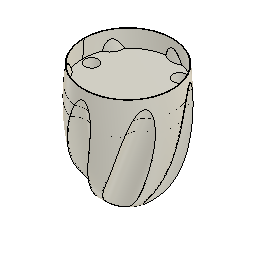
minlampshade twist tall v5 (Autodesk Fusion 360 design; units mm, degrees)
Autodesk Fusion 360 part; units mm, degrees
sketch "Sketch1" plane through (0, 0, 0) normal (0, 1, 0) x (1, 0, 0)
  line L0 (-68, -178) -> (68, -178)
  line L1 (68, -178) -> (68, 0)
  line L2 (-68, 0) -> (-68, -178)
  line L3 (-68, 0) -> (0, 0)
  line L4 (0, 0) -> (68, 0)
  spline S0 degree 5 poles (-68, -178) (-69.3462, -164.4991) (-71.1864, -138.6764) (-71.3876, -103.4793) (-66.4744, -63.741) (-51.543, -26.8671) (-28.7199, -3.9358) (0, 3.9151) (28.7199, -3.9358) (51.543, -26.8671) (66.4744, -63.741) (71.3876, -103.4793) (71.1864, -138.6764) (69.3462, -164.4991) (68, -178) knots 0 0 0 0 0 0 0.1 0.2 0.3 0.4 0.5 0.6 0.7 0.8 0.9 1 1 1 1 1 1
  line L5 (-10, 0) -> (10, 0)
  line L6 (-68, -8) -> (68, -8)
  line L7 (-27.7683, -8) -> (27.7683, -8)
  line L8 (27.7683, -8) -> (27.7683, 0)
  line L9 (27.7683, 0) -> (-27.7683, 0)
  line L10 (-27.7683, 0) -> (-27.7683, -8)
  line L11 (0, -178) -> (0, 0)
  dimension "d2" = 136
  dimension "d4" = 170
  dimension "d5" = 8
  dimension "d6" = 55.5365
  constraint horizontal L0
  constraint vertical L1
  constraint vertical L2
  constraint perpendicular L2 L3
  constraint perpendicular L1 L4
  constraint coincident L3.end L4.start
  constraint equal L3 L4
  constraint coincident L3 L4.start
  constraint midpoint L3.end L5
  constraint coincident L4 L5.end
  constraint coincident L2 L6.start
  constraint coincident L1 L6.end
  constraint perpendicular L1 L6
  constraint horizontal L7
  constraint vertical L8
  constraint horizontal L9
  constraint vertical L10
  constraint coincident L4 L8.end
  constraint coincident S0 L7.start
  constraint coincident L6 L7.start
  constraint coincident S0 L7.end
  constraint midpoint L0 L11.start
  measures "d2" distance of L0.start L0.end
  measures "d4" distance of L0 L6
  measures "d5" distance of L3 L6
  measures "d6" distance of L8 L10
revolve "Revolve1" add sketch "Sketch1" angle 360 about axis through (0, 0, 178) along (0, 0, -1) contours L0 L2 S0 L6 L7 L11 | L2 S0 makes body 1
sketch "Sketch2" plane through (0, 0, 8) normal (0, 0, -1) x (1, 0, 0)
  circle A0 centre (0, 0) radius 27.7683
  circle A1 centre (0, 0) radius 15
  dimension "d8" = 30
  constraint concentric A0 A1
  measures "d8" diameter of A1
extrude "Extrude1" cut sketch "Sketch2" against normal up to surface (170 mm away) contours A1 bodies 1
sketch "Sketch3" plane through (0, 0, 0) normal (0, 1, 0) x (1, 0, 0)
  line L0 (68, -178) -> (-68, -178)
  line L1 (27.7683, -8) -> (-27.7683, -8)
  line L2 (-80.8653, -168) -> (-118.4623, -154.3448)
  line L3 (-63.9824, -4.3448) -> (-26.3854, -18)
  line L4 (-80.8653, -168) -> (-26.3854, -18)
  line L5 (-118.4623, -154.3448) -> (-63.9824, -4.3448)
  line L6 (-99.6638, -161.1724) -> (-45.1839, -11.1724)
  spline S0 degree 5 poles (-68, -178) (-69.3462, -164.4991) (-71.1864, -138.6764) (-71.3876, -103.4793) (-66.4981, -63.9328) (-54.6444, -34.5268) (-42.2601, -18.6984) (-32.7386, -11.0612) (-27.7683, -8) knots 0 0 0 0 0 0 0.1 0.2 0.3 0.39807 0.39807 0.39807 0.39807 0.39807 0.39807
  spline S1 degree 5 poles (-68, -178) (-69.3462, -164.4991) (-71.1864, -138.6764) (-71.3876, -103.4793) (-66.4981, -63.9328) (-54.6444, -34.5268) (-42.2601, -18.6984) (-32.7386, -11.0612) (-27.7683, -8) knots 0 0 0 0 0 0 0.1 0.2 0.3 0.39807 0.39807 0.39807 0.39807 0.39807 0.39807
  dimension "d11" = 10
  dimension "d12" = 10
  dimension "d13" = 40
  constraint perpendicular L3 L4
  constraint perpendicular L3 L5
  constraint midpoint L2 L6.start
  constraint midpoint L3 L6.end
  constraint perpendicular L2 L4
  measures "d11" vertical distance of L1.end L3.end
  measures "d12" vertical distance of L0.end L2.start
  measures "d13" distance of L3.start L3.end
revolve "Revolve2" add sketch "Sketch3" angle 360 about axis through (-99.6638, 0, 161.1724) along (0.34138, 0, -0.939925) separate body contours L2 L3 L5 L6 makes body 2
move_face "OffsetFaces1" offset 80 1 faces at (-92.1555, -6.0867, 163.8994) on bodies 2
move_face "OffsetFaces2" offset 170 1 faces at (-49.8325, -0.9936, 9.484) on bodies 2
move_body "Move1" bodies 2 to x (0.998973, 0.044943, -0.005827) y (-0.04492, 0.998982, 0.004064) z (0.006004, -0.003798, 0.999975) at (-7.1443, 47.343, 78.4439)
pattern_circular "C-Pattern1" count 6 over 360 about axis through (0, 0, 8) along (0, 0, 1) of bodies 2 makes body 3 at (-88.7115, -70.6391, 180.2352) makes body 4 at (16.8195, -112.146, 180.2352) makes body 5 at (105.531, -41.5069, 180.2352) makes body 6 at (67.1377, 30.0885, 51.6608) makes body 7 at (13.7415, 99.1463, 190.0859)
combine "Combine1" operation cut target body 1 tool bodies 2 3 4 5 6 7
copy_body "CopyPasteBodies1" bodies 1 makes body 8
shell "Shell1" thickness 0.9 removed faces 2 at (14.9814, 0.7477, 121.3333) at (-50.0243, -4.1235, 178) on bodies 8
combine "Combine1'" operation cut target body 1 tool bodies 8 keep tools result as body 9 in component "Diffuser"
ref_plane "WorkPlane2" through (0, 0, 150) normal (0, 0, 1) x (1, 0, 0)
ref_plane "WorkPlane3" through (0, 0, 130) normal (0, 0, 1) x (1, 0, 0)
split "Split1" by plane through (0, 0, 150) normal (0, 0, 1) bodies 9 makes body 10 at (-31.1406, -38.6717, 178) in component "Diffuser"
split "Split2" by plane through (0, 0, 130) normal (0, 0, 1) bodies 9 makes body 11 at (-47.4733, 13.0915, 150) in component "Diffuser"
delete_body "RemoveBody1" bodies 9 in component "Diffuser"
delete_body "RemoveBody2" bodies 10 in component "Diffuser"
delete_face "DeleteFace1" 1 faces at (14.9255, 1.4935, 136.6667) on bodies 11 in component "Diffuser"
sketch "Sketch9" plane through (0, 0, 150) normal (0, 0, 1) x (-1, 0, 0)
  spline S0 degree 3 poles (64.5111, -25.0609) (65.3279, -22.9583) (66.0428, -20.8134) (68.3514, -12.5555) (69.2079, -6.2859) (69.2079, 0) knots -6.086236 -6.086236 -6.086236 -6.086236 -5.407133 -5.407133 -3.513875 -3.513875 -3.513875 -3.513875
  line L0 (0, 0) -> (-29.9329, -48.752) construction
  circle A0 centre (-29.9329, -48.752) radius 10
  spline S1 degree 3 poles (69.2079, 0) (69.2079, 2.6904) (69.051, 5.3837) (68.1977, 12.655) (67.2024, 17.1672) (65.7714, 21.5373) knots -3.513875 -3.513875 -3.513875 -3.513875 -2.703567 -2.703567 -1.317534 -1.317534 -1.317534 -1.317534
  ellipse E0 centre (74.9705, 41.7275) end of major axis (84.9657, 61.5383) minor radius 20.9 (53.9589, 43.3378) -> (65.7714, 21.5373) ccw
  spline S2 degree 3 poles (53.9589, 43.3378) (53.2294, 44.2461) (52.4767, 45.1363) (48.3094, 49.8193) (44.5062, 53.2443) (33.0406, 61.4757) (24.7634, 65.2512) (15.4097, 67.4732) (14.8224, 67.6046) (14.2338, 67.7283) knots -42.434116 -42.434116 -42.434116 -42.434116 -42.084235 -42.084235 -40.553499 -40.553499 -37.849932 -37.849932 -37.66929 -37.66929 -37.66929 -37.66929
  ellipse E1 centre (1.3482, 85.7902) end of major axis (-10.8109, 104.3516) minor radius 20.9 (-10.5521, 68.3987) -> (14.2338, 67.7283) ccw
  spline S3 degree 3 poles (-10.5521, 68.3987) (-10.6233, 68.3877) (-10.6944, 68.3766) (-19.6676, 66.9636) (-28.2109, 63.8364) (-41.7414, 55.6224) (-47.0037, 51.2496) (-51.5375, 46.191) knots -35.167956 -35.167956 -35.167956 -35.167956 -35.146366 -35.146366 -32.442799 -32.442799 -30.397785 -30.397785 -30.397785 -30.397785
  ellipse E2 centre (-73.6224, 44.0626) end of major axis (-95.7766, 42.8133) minor radius 20.9 (-64.5111, 25.0609) -> (-51.5375, 46.191) ccw
  spline S4 degree 3 poles (-64.5111, 25.0609) (-65.5466, 22.3952) (-66.4181, 19.6625) (-69.3161, 8.1379) (-69.7857, -0.9476) (-67.9288, -13.8382) (-67.014, -17.7424) (-65.7714, -21.5373) knots -27.89711 -27.89711 -27.89711 -27.89711 -27.035666 -27.035666 -24.332099 -24.332099 -23.128562 -23.128562 -23.128562 -23.128562
  ellipse E3 centre (-74.9705, -41.7275) end of major axis (-84.9657, -61.5383) minor radius 20.9 (-53.9589, -43.3378) -> (-65.7714, -21.5373) ccw
  spline S5 degree 3 poles (-53.9589, -43.3378) (-50.4196, -47.7445) (-46.3459, -51.7109) (-34.6426, -60.5874) (-26.4673, -64.5788) (-16.5889, -67.2012) (-15.414, -67.4803) (-14.2338, -67.7283) knots -20.628034 -20.628034 -20.628034 -20.628034 -18.924966 -18.924966 -16.221399 -16.221399 -15.858804 -15.858804 -15.858804 -15.858804
  ellipse E4 centre (-1.3482, -85.7902) end of major axis (10.8109, -104.3516) minor radius 20.9 (10.5521, -68.3987) -> (-14.2338, -67.7283) ccw
  spline S6 degree 3 poles (10.5521, -68.3987) (18.9222, -67.1074) (26.9894, -64.2898) (40.7946, -56.3972) (46.5961, -51.7044) (51.5375, -46.191) knots -13.357692 -13.357692 -13.357692 -13.357692 -10.814266 -10.814266 -8.587041 -8.587041 -8.587041 -8.587041
  ellipse E5 centre (73.6224, -44.0626) end of major axis (95.7766, -42.8133) minor radius 20.9 (64.5111, -25.0609) -> (51.5375, -46.191) ccw
  circle A1 centre (0, 0) radius 69.2079
  line L1 (-29.9329, -48.752) -> (-36.2117, -58.9783) construction
  line L2 (-14.2338, -67.7283) -> (-36.2117, -58.9783) construction
  line L3 (-36.2117, -58.9783) -> (-53.9589, -43.3378) construction
  dimension "d23" = 20
  dimension "d29" = 12
  constraint coincident L0.start A1.centre
  constraint coincident L0.end A0.centre
  constraint coincident S6.start A1
  constraint coincident S2.start A1
  constraint coincident S4.start A1
  constraint coincident A1 L1.end
  constraint coincident S5.end L2.start
  constraint coincident S5.start L3.end
  constraint equal L2 L3
  constraint collinear L0 L1
  measures "d23" diameter of A0
  measures "d29" distance of L0.end L1.end
extrude "Extrude1'" cut sketch "Sketch9" against normal through all contours A0 bodies 11 in component "Diffuser"
pattern_circular "C-Pattern1'" count 3 over 360 about axis through (0, 0, 1.75) along (0, 0, 1) of 1 faces at (19.9826, 49.7477, 143.3333) on bodies 11 in component "Diffuser"
sketch "Sketch10" plane through (0, 0, 150) normal (0, 0, 1) x (-1, 0, 0)
  circle A0 centre (-27.254, 50.2987) radius 10
  circle A1 centre (57.1869, -1.5467) radius 10
  spline S0 degree 3 poles (64.5111, -25.0609) (65.3279, -22.9583) (66.0428, -20.8134) (68.3514, -12.5555) (69.2079, -6.2859) (69.2079, 0) knots -6.086236 -6.086236 -6.086236 -6.086236 -5.407133 -5.407133 -3.513875 -3.513875 -3.513875 -3.513875
  circle A2 centre (0, 0) radius 67.8416
  spline S1 degree 3 poles (69.2079, 0) (69.2079, 2.6904) (69.051, 5.3837) (68.1977, 12.655) (67.2024, 17.1672) (65.7714, 21.5373) knots -3.513875 -3.513875 -3.513875 -3.513875 -2.703567 -2.703567 -1.317534 -1.317534 -1.317534 -1.317534
  ellipse E0 centre (74.9705, 41.7275) end of major axis (84.9657, 61.5383) minor radius 20.9 (53.9589, 43.3378) -> (65.7714, 21.5373) ccw
  spline S2 degree 3 poles (53.9589, 43.3378) (53.2294, 44.2461) (52.4767, 45.1363) (48.3094, 49.8193) (44.5062, 53.2443) (33.0406, 61.4757) (24.7634, 65.2512) (15.4097, 67.4732) (14.8224, 67.6046) (14.2338, 67.7283) knots -42.434116 -42.434116 -42.434116 -42.434116 -42.084235 -42.084235 -40.553499 -40.553499 -37.849932 -37.849932 -37.66929 -37.66929 -37.66929 -37.66929
  ellipse E1 centre (1.3482, 85.7902) end of major axis (-10.8109, 104.3516) minor radius 20.9 (-10.5521, 68.3987) -> (14.2338, 67.7283) ccw
  spline S3 degree 3 poles (-10.5521, 68.3987) (-10.6233, 68.3877) (-10.6944, 68.3766) (-19.6676, 66.9636) (-28.2109, 63.8364) (-41.7414, 55.6224) (-47.0037, 51.2496) (-51.5375, 46.191) knots -35.167956 -35.167956 -35.167956 -35.167956 -35.146366 -35.146366 -32.442799 -32.442799 -30.397785 -30.397785 -30.397785 -30.397785
  ellipse E2 centre (-73.6224, 44.0626) end of major axis (-95.7766, 42.8133) minor radius 20.9 (-64.5111, 25.0609) -> (-51.5375, 46.191) ccw
  spline S4 degree 3 poles (-64.5111, 25.0609) (-65.5466, 22.3952) (-66.4181, 19.6625) (-69.3161, 8.1379) (-69.7857, -0.9476) (-67.9288, -13.8382) (-67.014, -17.7424) (-65.7714, -21.5373) knots -27.89711 -27.89711 -27.89711 -27.89711 -27.035666 -27.035666 -24.332099 -24.332099 -23.128562 -23.128562 -23.128562 -23.128562
  ellipse E3 centre (-74.9705, -41.7275) end of major axis (-84.9657, -61.5383) minor radius 20.9 (-53.9589, -43.3378) -> (-65.7714, -21.5373) ccw
  spline S5 degree 3 poles (-53.9589, -43.3378) (-50.4196, -47.7445) (-46.3459, -51.7109) (-34.6426, -60.5874) (-26.4673, -64.5788) (-16.5889, -67.2012) (-15.414, -67.4803) (-14.2338, -67.7283) knots -20.628034 -20.628034 -20.628034 -20.628034 -18.924966 -18.924966 -16.221399 -16.221399 -15.858804 -15.858804 -15.858804 -15.858804
  ellipse E4 centre (-1.3482, -85.7902) end of major axis (10.8109, -104.3516) minor radius 20.9 (10.5521, -68.3987) -> (-14.2338, -67.7283) ccw
  spline S6 degree 3 poles (10.5521, -68.3987) (18.9222, -67.1074) (26.9894, -64.2898) (40.7946, -56.3972) (46.5961, -51.7044) (51.5375, -46.191) knots -13.357692 -13.357692 -13.357692 -13.357692 -10.814266 -10.814266 -8.587041 -8.587041 -8.587041 -8.587041
  ellipse E5 centre (73.6224, -44.0626) end of major axis (95.7766, -42.8133) minor radius 20.9 (64.5111, -25.0609) -> (51.5375, -46.191) ccw
  circle A3 centre (-29.9329, -48.752) radius 10
  dimension "d28" = 135.6832
  constraint coincident A2.centre origin
  measures "d28" diameter of A2
component "Diffuser" placed x (1, 0, 0) y (0, 1, 0) z (0, 0, 1) at (0, 0, 0)
hidden bodies 1
named bodies: "Lampshade", "Lampshade Shell", "Lampshade (1)", "Diffuser"
